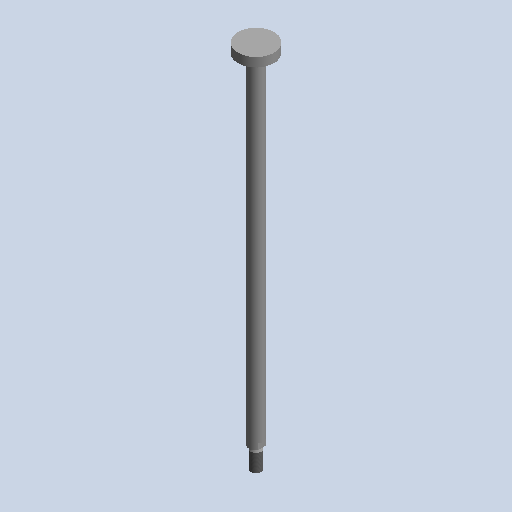
# Autodesk Inventor part: 193993 DSNU-40-300-P---(A---00--0-KS)
Saved by Autodesk Inventor 2022 (Build 260153000, 153)
## iProperties
Part Number: 193993 DSNU-40-300-P---(A---00--0-KS)
Material: Generic
Catalog Web Link: www.cadenas.de
Description: DSNU---(KS)-Standard cylinder
Vendor: FESTO
Document SubType Name: Modeling
Designer: partserver
Manufacturer: FESTO
Mass: 90.6613 g
Surface Area: 235.619 cm^2
Volume: 90.6613 cm^3
Density: 1 g/cm^3
Appearance: PSOLRGB-192-192-192
Category: PARTsolutions
Company: FESTO
PSOL_IDENT_0: {$CADENAS_DATA\23d-libs\festo\parts\d\dsnu\parts\dsnu_metric_ks.prj},256 {VTYP=3D},{NB=193993 DSNU-4
PSOL_IDENT_1: 0-300-P---(A---00--0-KS)},{LINA=193993 DSNU-40-300-P},{NN=DSNU---(KS)},{DATE=23.06.2020 07:36:01},{G
PSOL_IDENT_2: EOMDATE=06.03.2020 09:03:14},{VERSION=},{LINEID=80},{WBVAR=TNR,HUB,DA,PE,ZD,VS,KA,K2A,K6,K3,K5,K8,KP
PSOL_IDENT_3: },{WBNUMERIC=HUB,K2A,K6,K8}  {NB=193993 DSNU-40-300-P---(A---00--0-KS)},{LINA=193993 DSNU-40-300-P},
PSOL_IDENT_4: {KT=DUMMY},{TNR=193993},{TYP=DSNU-40},{DSNU=METRIC},{KDM=40},{HUB=300},{DA=P},{DA1='P','PPV','PPS'},
PSOL_IDENT_5: {PE=A},{ZD=-},{VS=-},{VSALG='-','Q'},{KA=-},{KAALG='-','S2'},{K2A=0},{K6=0},{K3=-},{K31='-','K3'},{K
PSOL_IDENT_6: 5=-},{K51='-','M12'},{K8=0},{KP=-},{KPALG='-','KP'},{A1=35},{A2=500},{A3=8},{A4=70.5},{AB=38},{AM=24
PSOL_IDENT_7: },{B=38},{BB=4},{BE=M38x1,5},{BENDM=38.000},{BEKDM=36.160},{BEP=1.500},{BS=9.0},{B1=54},{B2=13},{B3=
PSOL_IDENT_8: 38},{B4=12},{B5=32.0},{B6=14},{B7=4},{CD=12},{D=46},{D1=38},{D2=16},{D3=41.6},{D4=12.0},{D5=42.0},{D
PSOL_IDENT_9: 6=50},{D7=38},{EE=G1/4},{EENDM=13.157},{EEKDM=11.445},{EW=18},{F=42},{FF=M5},{FFNDM=5.000},{FFKDM=4.
PSOL_IDENT_10: 019},{F1=24},{H=48},{H1=7},{KK=M12x1.25},{KKNDM=12.000},{KKKDM=0.000},{KKP=1.250},{K1=M8},{K1NDM=8.0
PSOL_IDENT_11: 00},{K1KDM=6.466},{K2=3.0},{KV=0},{KW=10},{L=15},{LH=15.0},{LK=18.0},{L1=153.6},{L2=84.6},{L3=12.0},
PSOL_IDENT_12: {L4=30.0},{L5=27},{L6=63},{L7=33},{L8=25.0},{L9=29.0},{L10=104.6},{L11=116.6},{L12=77.6},{L13=162.6}
PSOL_IDENT_13: ,{ST=9.0},{SW=13},{T=12},{WH=39},{X=3.3},{XC=139.6},{K1KP=56},{K2KP=M8},{K2KPNDM=8.000},{K3KP=18},{K
PSOL_IDENT_14: 4KP=28.0},{K5KP=89.0},{K6KP=6.8},{K7KP=24},{K8KP=36.0},{K9KP=17.0},{K10KP=7.0},{K11KP=20},{K12KP=G1/
PSOL_IDENT_15: 8},{K12KPNDM=9.728},{K13KP=69},{ZRSTART=55},{MHL=45.000},{ZRL=34.6},{C=21.200},{WHX=12.000},{LD1=35.
PSOL_IDENT_16: 800},{LD2=35.700},{AD1=14.000},{AD2=12.000},{AD3=10.500},{AD4=9.000},{AD5=12.500},{MH1=11.000},{MH2=
PSOL_IDENT_17: 2.600},{MH3=15.200},{KP1=34.000},{KP2=30.000},{KP3=24.000},{KP4=25.000},{KP5=45.000},{KPC=22.000},{K
PSOL_IDENT_18: PF=3.000},{KPG=22.000},{KPH=83.000},{KPJ=23.500},{KPK=17.000},{KPL=4.500},{KPR3=1.000},{KPR=23.000},
PSOL_IDENT_19: {KPS=20.500},{MLD1=55.000},{MLD2=48.000},{MLD3=5.000},{MLL1=16.000},{KL1=76},{KKC=10.2},{KKD=1.5},{K
PSOL_IDENT_20: KF=0.6},{SWL=6.500},{K3L=8.400},{HUB1=300},{FDTXF31=5.000},{FDTB31=6.000}
NB: 193993 DSNU-40-300-P---(A---00--0-KS)
NN: DSNU---(KS)
NT: Standard cylinder
NBSYN: $TNR. $TYP.-$HUB1.-$DA.---($PE.$ZD.$VS.$KA.$K2A.$K6.$K3.$K5.$K8.$KP.KS)
LINA: 193993 DSNU-40-300-P
CATALOG: Festo
TNR: 193993
TYP: DSNU-40
DSNU: METRIC
KDM: 40
HUB: 300
DA: P
DA1: 'P','PPV','PPS'
PE: A
ZD: -
VS: -
KA: -
K2A: 0
K6: 0
K3: -
K31: '-','K3'
K5: -
K51: '-','M12'
K8: 0
KP: -
A1: 35
A2: 500
A3: 8
A4: 70.5
AB: 38
AM: 24
B: 38
BB: 4
BE: M38x1,5
BENDM: 38
BEKDM: 36.16
BEP: 1.5
BS: 9
B1: 54
B2: 13
B3: 38
B4: 12
B5: 32
B6: 14
B7: 4
CD: 12
D: 46
D1: 38
D2: 16
D3: 41.6
D4: 12
D5: 42
D6: 50
D7: 38
EE: G1/4
EENDM: 13.157
EEKDM: 11.445
EW: 18
F: 42
FF: M5
FFNDM: 5
FFKDM: 4.019
F1: 24
H: 48
H1: 7
KK: M12x1.25
KKNDM: 12
KKKDM: 0
KKP: 1.25
K1: M8
K1NDM: 8
K1KDM: 6.466
K2: 3
KV: 0
KW: 10
L: 15
LH: 15
LK: 18
L3: 12
L4: 30
L5: 27
L6: 63
L7: 33
L8: 25
L9: 29
L13: 162.6
ST: 9
SW: 13
T: 12
X: 3.3
K1KP: 56
K2KP: M8
K2KPNDM: 8
K3KP: 18
K4KP: 28
K5KP: 89
K6KP: 6.8
K7KP: 24
K8KP: 36
K9KP: 17
K10KP: 7
K11KP: 20
K12KP: G1/8
K12KPNDM: 9.728
K13KP: 69
MHL: 45
C: 21.2
WHX: 12
LD1: 35.8
LD2: 35.7
AD1: 14
AD2: 12
AD3: 10.5
AD4: 9
AD5: 12.5
MH1: 11
MH2: 2.6
MH3: 15.2
KP1: 34
KP2: 30
KP3: 24
KP4: 25
KP5: 45
KPC: 22
KPF: 3
KPG: 22
KPH: 83
KPJ: 23.5
KPK: 17
KPL: 4.5
KPR3: 1
KPR: 23
KPS: 20.5
MLD1: 55
MLD2: 48
MLD3: 5
MLL1: 16
SWL: 6.5
K3L: 8.4
FDTXF31: 5
FDTB31: 6
SUPPLIER: FESTO
ARTICLENO: 193993 DSNU-40-300-P---(A---00--0-KS)
BOMINFO: 193993 DSNU-40-300-P
CREATOR: CADENAS GmbH
Title: 193993 DSNU-40-300-P
Author: Cadenas PARTsolutions
Comments: Standard cylinder
Autodesk Inventor part; units mm, degrees
sketch "Sketch_2" plane through (0, 0, 0) normal (1, 0, 0) x (0, 1, 0)
  line L0 (0, -377) -> (0, 9)
  line L1 (0, 9) -> (8, 9)
  line L2 (8, 9) -> (8, -367)
  line L3 (8, -367) -> (20, -367)
  line L4 (20, -367) -> (20, -377)
  line L5 (20, -377) -> (0, -377)
  line L6 (0, -377) -> (0, 9)
  constraints: 14 end point
revolve "Revolution1" add sketch "Sketch_2" angle 360 about axis through (0, 0, -377) along (0, 0, -1)
sketch "Sketch_6" plane through (0, 0, 0) normal (1, 0, 0) x (0, 1, 0)
  line L0 (0, 8) -> (0, 33)
  line L1 (0, 33) -> (5.233, 33)
  line L2 (5.233, 33) -> (6, 32.233)
  line L3 (6, 32.233) -> (6, 12.9727)
  line L4 (6, 12.9727) -> (5.1362, 10.5994)
  arc A0 (5.1362, 10.5994) -> (5.1, 10.3942) centre (5.7, 10.3942) ccw
  line L5 (5.1, 10.3942) -> (5.1, 9.6)
  arc A1 (5.1, 9.6) -> (5.7, 9) centre (5.7, 9.6) ccw
  line L6 (5.7, 9) -> (6, 9)
  line L7 (6, 9) -> (6, 8)
  line L8 (6, 8) -> (0, 8)
  line L9 (0, 8) -> (0, 33)
  constraints: 20 end point, 4 point on circle, 2 centre point
revolve "Revolution2" add sketch "Sketch_6" angle 360 about axis through (0, 0, 8) along (0, 0, -1)
thread "Thread1" size "M12x1.25" class "6g" standard "ISO Metric profile" full length
sketch "Sketch_7" plane through (0, 0, 2.5) normal (0, 0, 1) x (1, 0, 0)
  line L0 (-13, 26) -> (-13, -13)
  line L1 (-13, -13) -> (-6.5, -13)
  line L2 (-6.5, -13) -> (-6.5, 13)
  line L3 (-6.5, 13) -> (6.5, 13)
  line L4 (6.5, 13) -> (6.5, -13)
  line L5 (6.5, -13) -> (13, -13)
  line L6 (13, -13) -> (13, 26)
  line L7 (13, 26) -> (-13, 26)
  constraints: 16 end point
extrude "Extrusion1" cut sketch "Sketch_7" along normal blind 7.5
ref_plane "FDT_KSAUFSATZ_XY" through (0, 0, 20) normal (0, 0, 1) x (-1, 0, 0)
ref_plane "FDT_KSAUFSATZ_YZ" through (0, 0, 20) normal (-1, 0, 0) x (0, -1, 0)
ref_plane "FDT_KSAUFSATZ_ZX" through (0, 0, 20) normal (0, -1, 0) x (0, 0, 1)
ref_plane "FDT_NUT_XY" through (0, 0, 20) normal (0, 0, 1) x (-1, 0, 0)
ref_plane "FDT_NUT_YZ" through (0, 0, 20) normal (-1, 0, 0) x (0, -1, 0)
ref_plane "FDT_NUT_ZX" through (0, 0, 20) normal (0, -1, 0) x (0, 0, 1)
ref_plane "KS_XY" through (0, 0, 0) normal (0, 0, -1) x (1, 0, 0)
ref_plane "KS_YZ" through (0, 0, 0) normal (1, 0, 0) x (0, -1, 0)
ref_plane "KS_ZX" through (0, 0, 0) normal (0, -1, 0) x (0, 0, -1)
ref_plane "NUT1_XY" through (0, 0, 24) normal (0, 0, 1) x (1, 0, 0)
ref_plane "NUT1_YZ" through (0, 0, 24) normal (1, 0, 0) x (0, 1, 0)
ref_plane "NUT1_ZX" through (0, 0, 24) normal (0, 1, 0) x (0, 0, 1)
body "Solid1"
